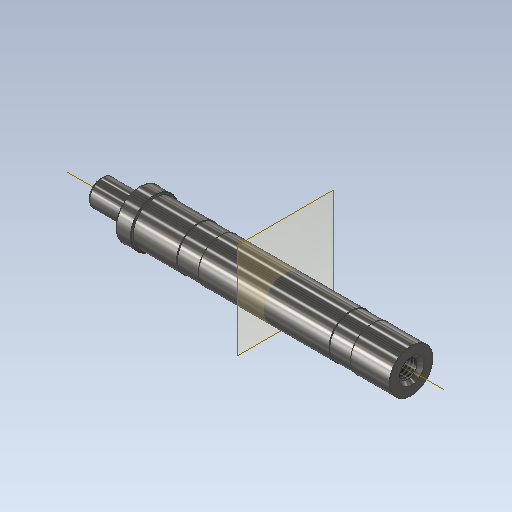
# Autodesk Inventor part: Shoulder_Joint_Yawn_Shaft
Saved by Autodesk Inventor 2021.4 (Build 254397000, 397)
## iProperties
Created: 2020-05-04
Part Number: Shoulder_Joint_Yawn_Shaft
Material: Stahl, hochfest, niedrig legiert
Document SubType Name: Modeling
Designer: Alex
Density: 7.85 g/cm^3
Appearance: Stahl - poliert
Mass: 39.0682 g
Surface Area: 25.1118 cm^2
Volume: 4.97684 cm^3
YawnFixation_Width: 30,200 mm
YawnShaft_Diameter: 10,000 mm
Author: Alex
Autodesk Inventor part; units mm, degrees
ref_plane "YZ Plane" through (0, 0, 0) normal (1, 0, 0) x (0, 1, 0)
ref_plane "XZ Plane" through (0, 0, 0) normal (0, 1, 0) x (-1, 0, 0)
ref_plane "XY Plane" through (0, 0, 0) normal (0, 0, 1) x (1, 0, 0)
sketch "Skizze1" plane through (0, 0, 0) normal (0, 0, 1) x (1, 0, 0)
  line L0 (0, 5.5) -> (3.5, 5.5)
  line L1 (3.5, 5.5) -> (3.5, 5)
  line L2 (3.5, 5) -> (13.5, 5)
  line L3 (13.5, 5) -> (13.5, 5)
  line L4 (53.5, 5) -> (53.5, 5)
  line L5 (53.5, 5) -> (62.5, 5)
  line L6 (62.5, 0) -> (0, 0)
  line L7 (0, 3) -> (0, 5.5)
  arc A0 (13.5, 5) -> (13.6, 4.9) centre (13.6, 5) ccw
  arc A1 (53.4, 4.9) -> (53.5, 5) centre (53.4, 5) ccw
  line L8 (18.5, 5) -> (18.5, 5)
  line L9 (18.5, 5) -> (48.5, 5)
  line L10 (48.5, 5) -> (48.5, 5)
  line L11 (13.6, 4.9) -> (18.4, 4.9)
  line L12 (48.6, 4.9) -> (53.4, 4.9)
  arc A2 (18.4, 4.9) -> (18.5, 5) centre (18.4, 5) ccw
  arc A3 (48.5, 5) -> (48.6, 4.9) centre (48.6, 5) ccw
  line L13 (62.5, 5) -> (62.5, 0)
  line L14 (0, 3) -> (-9, 3)
  line L15 (-9, 3) -> (-9, 0)
  line L16 (-9, 0) -> (0, 0)
  line L17 (0, -16.1) -> (0, 16.1) construction
  line L18 (-0.5, -11.5) -> (-0.5, 11.5) projected
  point P0 (33.5, 5)
  dimension "d0" = 11
  dimension "d1" = 3.5
  dimension "YawnShaft_Diameter" = 10
  dimension "d4" = 13.5
  dimension "d7" = 0.1
  dimension "d13" = 9.8
  dimension "d14" = 10
  dimension "d16" = 30
  dimension "d17" = 40
  dimension "d18" = 5
  dimension "d19" = 0.1
  dimension "d49" = 5
  dimension "d51" = 62.5
  dimension "d52" = 59
  dimension "d54" = 30
  dimension "d57" = 6
  dimension "d63" = 8.5
  dimension "YawnFixation_Width" = 30.2
  constraints: 34 end point, 16 perpendicular, 10 tangent, 8 point on circle, 4 centre point, 2 equal radius, 2 parallel, 2 point on line, 1 collinear, 1 horizontal, 1 midpoint
  measures "d0" diameter of L0 L6
  measures "d1" distance between parallel lines of L1 L7
  measures "YawnShaft_Diameter" diameter of L2 L6
  measures "d4" distance between parallel lines of L3 L7
  measures "d7" radius of A0
  measures "d13" diameter of L11 L6
  measures "d14" diameter of L9 L6
  measures "d16" distance between parallel lines of L10 L8
  measures "d17" distance of L4.start L3.end
  measures "d18" distance from line of L8 L2.end
  measures "d19" radius of A2
  measures "d49" distance of L4.end L9.end
  measures "d51" distance between parallel lines of L13 L7
  measures "d52" distance between parallel lines of L13 L1
  measures "d54" distance from line of L1 point (33.5, 5)
  measures "d57" diameter of L14 L16
  measures "d63" distance between parallel lines of L18 L15
  measures "YawnFixation_Width" distance of A3.centre A2.centre
revolve "Grundprofil" add sketch "Skizze1" angle 360 about axis through (62.5, 0, 0) along (-1, 0, 0)
chamfer "Entgraten 0,1mm" distance 0.1 angle 45 3 edges at (0, -5.5, 0) (3.5, -5.5, 0) (62.5, -5, 0)
sketch "Skizze4" plane through (62.5, 0, 0) normal (1, 0, 0) x (0, 0, -1)
  point P0 (0, 0)
  point P1 (0, 0)
  constraints: 1 coincident
hole "Gewinde_Keine_ISO Metrisches Profil_5_Winkel" at (62.5, 0, 0) direction (-1, 0, 0) diameter 4.134 depth 15 tip angle 118 thread size "M5x0.8" class "6H" standard "ISO Metric profile"
chamfer "Gewindefase 0,8mm" distance 0.8 angle 45 1 edges at (62.5, 0, 2.067)
fillet "Kerbwirkungsreduktion 0,5mm" radius 0.5 1 edges at (0, -3, 0)
chamfer "Encoderschaft Fase 0,5mm" distance 0.5 angle 45 1 edges at (-9, -3, 0)
ref_plane "Work Plane1" through (33.5, 5, 0) normal (1, 0, 0) x (0, 1, 0)
equation "\"d7\" = d19"
equation "\"d18\" = -0.5 * d16 + 0.5 * d17"
equation "\"d19\" = -0.5 * d13 + 0.5 * YawnShaft_Diameter"
